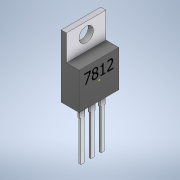
# Autodesk Inventor part: 7805
Saved by Autodesk Inventor 2020 (Build 240168000, 168)
## iProperties
Created: 2021-10-19
Part Number: 7805
Material: Genérico
Document SubType Name: Modeling
Designer: DANIEL
Density: 1 g/cm^3
Appearance: Valor por defecto
Author: DANIEL
Autodesk Inventor part; units mm, degrees
ref_plane "YZ Plane" through (0, 0, 0) normal (1, 0, 0) x (0, 1, 0)
ref_plane "XZ Plane" through (0, 0, 0) normal (0, 1, 0) x (-1, 0, 0)
ref_plane "XY Plane" through (0, 0, 0) normal (0, 0, 1) x (1, 0, 0)
sketch "Boceto1" plane through (0, 0, 0) normal (0, 1, 0) x (-1, 0, 0)
  line L0 (2.25, 4.95) -> (-2.25, 4.95)
  line L1 (-2.25, 4.95) -> (-2.25, -4.95)
  line L2 (-2.25, -4.95) -> (2.25, -4.95)
  line L3 (2.25, -4.95) -> (2.25, 4.95)
  point P0 (0, 0)
  dimension "d0" = 4.5
  dimension "d1" = 9.9
  dimension "d2" = 4.95
  dimension "d3" = 2.25
  constraints: 8 end point, 2 parallel, 1 horizontal, 1 perpendicular
  measures "d0" distance between parallel lines of L1 L3
  measures "d1" distance between parallel lines of L0 L2
  measures "d2" distance from line of L0 point (0, 0)
  measures "d3" distance from line of L3 point (0, 0)
extrude "Extrusión1" add sketch "Boceto1" along normal mid plane 9.2
sketch "Boceto2" plane through (0, 4.6, 0) normal (0, 1, 0) x (1, 0, 0)
  line L0 (2.25, 4.95) -> (-2.25, 4.95) projected
  line L1 (-2.25, 4.95) -> (-2.25, -4.95) projected
  line L2 (-2.25, -4.95) -> (2.25, -4.95) projected
  line L3 (2.25, -4.95) -> (2.25, 4.95) projected
  line L4 (2.25, 4.95) -> (-2.25, 4.95) projected
  line L5 (-2.25, -4.95) -> (-0.95, -4.95)
  line L6 (-0.95, -4.95) -> (-0.95, 4.95)
  line L7 (-0.95, 4.95) -> (-2.25, 4.95)
  line L8 (-2.25, 4.95) -> (-2.25, -4.95)
  point P0 (0, 0)
  point P1 (-0.95, 4.95)
  dimension "d6" = 1.3
  constraints: 8 end point, 2 parallel, 1 horizontal, 1 perpendicular, 1 point on line
  measures "d6" distance of L7.end L6.end
extrude "Extrusión2" add sketch "Boceto2" along normal blind 6.5 contours L6 L2 L1 L0
sketch "Boceto3" plane through (-0.95, 4.6, 4.95) normal (1, 0, 0) x (0, 0, -1)
  line L0 (9.9, 0) -> (0, 0) projected
  line L1 (9.9, 0) -> (9.9, 6.5) projected
  line L2 (0, 6.5) -> (9.9, 6.5) projected
  line L3 (0, 0) -> (0, 6.5) projected
  circle A0 centre (4.95, 3.7) radius 1.8
  point P0 (4.95, -4.6)
  dimension "d9" = 3.6
  dimension "d10" = 4.95
  dimension "d11" = 3.7
  constraints: 1 centre point
  measures "d9" diameter of A0
  measures "d10" distance from line of L3 A0.centre
  measures "d11" distance from line of A0.centre L0
extrude "Extrusión3" cut sketch "Boceto3" against normal blind 6.5 contours A0
sketch "Boceto4" plane through (0, -4.6, 0) normal (0, -1, 0) x (1, 0, 0)
  line L0 (-2.25, -4.95) -> (2.25, -4.95) projected
  line L1 (2.25, -4.95) -> (2.25, 4.95) projected
  line L2 (2.25, 4.95) -> (-2.25, 4.95) projected
  line L3 (-2.25, 4.95) -> (-2.25, -4.95) projected
  line L4 (0.65, 3.175) -> (0.15, 3.175)
  line L5 (0.15, 3.175) -> (0.15, 1.905)
  line L6 (0.15, 1.905) -> (0.65, 1.905)
  line L7 (0.65, 1.905) -> (0.65, 3.175)
  line L8 (0.65, 0.635) -> (0.15, 0.635)
  line L9 (0.15, 0.635) -> (0.15, -0.635)
  line L10 (0.15, -0.635) -> (0.65, -0.635)
  line L11 (0.65, -0.635) -> (0.65, 0.635)
  line L12 (0.65, -1.905) -> (0.15, -1.905)
  line L13 (0.15, -1.905) -> (0.15, -3.175)
  line L14 (0.15, -3.175) -> (0.65, -3.175)
  line L15 (0.65, -3.175) -> (0.65, -1.905)
  point P0 (0, 0)
  dimension "d14" = 1.27
  dimension "d15" = 1.27
  dimension "d16" = 1.27
  dimension "d17" = 0.5
  dimension "d18" = 0.5
  dimension "d19" = 0.5
  dimension "d20" = 1.27
  dimension "d21" = 1.27
  dimension "d22" = 4.315
  dimension "d23" = 2.4
  constraints: 24 end point, 6 parallel, 3 horizontal, 3 perpendicular, 3 point on line
  measures "d14" distance between parallel lines of L6 L4
  measures "d15" distance between parallel lines of L10 L8
  measures "d16" distance between parallel lines of L14 L12
  measures "d17" distance between parallel lines of L5 L7
  measures "d18" distance between parallel lines of L9 L11
  measures "d19" distance between parallel lines of L13 L15
  measures "d20" distance between parallel lines of L8 L6
  measures "d21" distance between parallel lines of L10 L12
  measures "d22" distance between parallel lines of L8 L2
  measures "d23" distance between parallel lines of L5 L3
extrude "Extrusión4" add sketch "Boceto4" along normal blind 3 contours L7 L6 L5 L4 | L11 L10 L9 L8 | L15 L14 L13 L12
sketch "Boceto5" plane through (0, -7.6, 0) normal (0, -1, 0) x (1, 0, 0)
  line L0 (0.15, 3.175) -> (0.15, 1.905) projected
  line L1 (0.15, 1.905) -> (0.65, 1.905) projected
  line L2 (0.65, 1.905) -> (0.65, 3.175) projected
  line L3 (0.65, 3.175) -> (0.15, 3.175) projected
  line L4 (0.15, 0.635) -> (0.15, -0.635) projected
  line L5 (0.15, -0.635) -> (0.65, -0.635) projected
  line L6 (0.65, -0.635) -> (0.65, 0.635) projected
  line L7 (0.65, 0.635) -> (0.15, 0.635) projected
  line L8 (0.65, -1.905) -> (0.15, -1.905) projected
  line L9 (0.15, -1.905) -> (0.15, -3.175) projected
  line L10 (0.15, -3.175) -> (0.65, -3.175) projected
  line L11 (0.65, -3.175) -> (0.65, -1.905) projected
  line L12 (0.15, 1.905) -> (0.15, 3.175) projected
  line L13 (0.65, 2.94) -> (0.15, 2.94)
  line L14 (0.15, 2.94) -> (0.15, 2.14)
  line L15 (0.15, 2.14) -> (0.65, 2.14)
  line L16 (0.65, 2.14) -> (0.65, 2.94)
  line L17 (0.15, 0.635) -> (0.15, -0.635) projected
  line L18 (0.65, 0.4) -> (0.15, 0.4)
  line L19 (0.15, 0.4) -> (0.15, -0.4)
  line L20 (0.15, -0.4) -> (0.65, -0.4)
  line L21 (0.65, -0.4) -> (0.65, 0.4)
  line L22 (0.65, -1.905) -> (0.65, -3.175) projected
  line L23 (0.15, -3.175) -> (0.15, -1.905) projected
  line L24 (0.65, -2.14) -> (0.15, -2.14)
  line L25 (0.15, -2.14) -> (0.15, -2.94)
  line L26 (0.15, -2.94) -> (0.65, -2.94)
  line L27 (0.65, -2.94) -> (0.65, -2.14)
  point P0 (0, 0)
  point P1 (0.15, -2.14)
  dimension "d26" = 0.8
  dimension "d27" = 0.8
  dimension "d28" = 0.8
  dimension "d29" = 0.235
  dimension "d30" = 0.235
  dimension "d31" = 0.235
  constraints: 24 end point, 6 parallel, 6 point on line, 3 horizontal, 3 perpendicular
  measures "d26" distance of L14.end L13.end
  measures "d27" distance of L19.end L18.end
  measures "d28" distance of L25.end L24.end
  measures "d29" distance between parallel lines of L13 L3
  measures "d30" distance between parallel lines of L7 L18
  measures "d31" distance between parallel lines of L24 L8
extrude "Extrusión5" add sketch "Boceto5" along normal blind 10.08 contours L13 L2 L15 L0 | L18 L6 L20 L4 | L11 L26 L9 L24
sketch "Boceto6" plane through (2.25, -4.6, -4.95) normal (1, 0, 0) x (0, 0, -1)
  line L0 (-8.7824, 7.8194) -> (-0.868, 7.8194) construction
  line L1 (-0.868, 7.8194) -> (-0.868, 3.7441) construction
  line L2 (-0.868, 3.7441) -> (-8.7824, 3.7441) construction
  line L3 (-8.7824, 3.7441) -> (-8.7824, 7.8194) construction
  point P0 (-4.95, 4.6)
  constraints: 2 other
